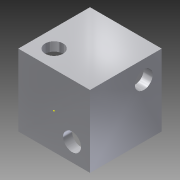
# Autodesk Inventor part: Corner
Saved by Autodesk Inventor 2015 SP1 (Build 190203100, 203)
## iProperties
Created: 2015-06-22
Part Number: Corner
Material: Aluminum 6061
Document SubType Name: Modeling
Designer: Kartikye
Density: 2.7 g/cm^3
Appearance: Aluminum - Flat
Author: Kartikye
Autodesk Inventor part; units mm, degrees
ref_plane "YZ Plane" through (0, 0, 0) normal (1, 0, 0) x (0, 1, 0)
ref_plane "XZ Plane" through (0, 0, 0) normal (0, 1, 0) x (-1, 0, 0)
ref_plane "XY Plane" through (0, 0, 0) normal (0, 0, 1) x (1, 0, 0)
sketch "Sketch1" plane through (0, 0, 0) normal (0, 1, 0) x (-1, 0, 0)
  point P0 (0, 0)
sketch "Sketch2" plane through (0, 0, 0) normal (0, 1, 0) x (-1, 0, 0)
  line L0 (-4, 4) -> (4, 4)
  line L1 (4, 4) -> (4, -4)
  line L2 (4, -4) -> (-4, -4)
  line L3 (-4, -4) -> (-4, 4)
  line L4 (-4, 4) -> (4, -4) construction
  line L5 (4, 4) -> (-4, -4) construction
  point P0 (0, 0)
  dimension "d0" = 8
  dimension "d1" = 8
  constraints: 12 end point, 2 midpoint, 2 parallel, 1 horizontal, 1 perpendicular
  measures "d0" distance of L1.end L2.end
  measures "d1" distance of L0.end L1.end
extrude "Extrusion1" add sketch "Sketch2" along normal blind 8
sketch "Sketch3" plane through (-4, 0, -4) normal (-1, 0, 0) x (0, 0, 1)
  line L0 (0, 1) -> (7, 1)
  line L1 (7, 1) -> (7, 7)
  line L2 (7, 7) -> (0, 7)
  line L3 (0, 7) -> (0, 1)
  line L4 (8, 0) -> (0, 0) projected
  line L5 (0, 0) -> (0, 8) projected
  point P0 (4, 0)
  dimension "d4" = 7
  dimension "d5" = 6
  dimension "d6" = 1
  dimension "d7" = 0
  constraints: 8 end point, 2 parallel, 1 horizontal, 1 perpendicular
  measures "d4" distance of L2.end L1.end
  measures "d5" distance of L1.end L0.end
  measures "d6" distance between parallel lines of L4 L0
  measures "d7" distance between parallel lines of L5 L3
extrude "Extrusion2" cut sketch "Sketch3" against normal blind 7
sketch "Sketch4" plane through (-4, 0, 4) normal (0, 0, 1) x (1, 0, 0)
  circle A0 centre (2, 2) radius 1
  line L0 (8, 0) -> (0, 0) projected
  line L1 (8, 0) -> (8, 8) projected
  point P0 (4, 0)
  dimension "d10" = 2
  dimension "d11" = 2
  dimension "d12" = 6
  constraints: 1 centre point
  measures "d10" diameter of A0
  measures "d11" distance from line of A0.centre L0
  measures "d12" distance from line of L1 A0.centre
sketch "Sketch5" plane through (4, 0, 4) normal (1, 0, 0) x (0, 0, -1)
  circle A0 centre (2, 6) radius 1
  line L0 (0, 0) -> (0, 8) projected
  line L1 (8, 0) -> (0, 0) projected
  point P0 (4, 0)
  dimension "d13" = 2
  dimension "d14" = 2
  dimension "d15" = 6
  constraints: 1 centre point
  measures "d13" diameter of A0
  measures "d14" distance from line of L0 A0.centre
  measures "d15" distance from line of L1 A0.centre
sketch "Sketch6" plane through (0, 0, 0) normal (0, -1, 0) x (1, 0, 0)
  circle A0 centre (2, -2) radius 1
  line L0 (4, 4) -> (-4, 4) projected
  line L1 (4, -4) -> (4, 4) projected
  point P0 (0, 0)
  dimension "d16" = 2
  dimension "d17" = 6
  dimension "d18" = 2
  constraints: 1 centre point
  measures "d16" diameter of A0
  measures "d17" distance from line of L0 A0.centre
  measures "d18" distance from line of L1 A0.centre
extrude "Extrusion3" cut sketch "Sketch6" against normal blind 1
extrude "Extrusion4" cut sketch "Sketch5" against normal blind 1
extrude "Extrusion5" cut sketch "Sketch4" against normal blind 1
sketch "Sketch7" plane through (0, 8, 0) normal (0, 1, 0) x (1, 0, 0)
  circle A0 centre (0, 0) radius 1
  line L0 (4, 4) -> (-4, 4) projected
  line L1 (-4, 4) -> (-4, -4) projected
  dimension "d25" = 2
  dimension "d26" = 4
  dimension "d27" = 4
  constraints: 1 centre point
  measures "d25" diameter of A0
  measures "d26" distance from line of A0.centre L0
  measures "d27" distance from line of L1 A0.centre
extrude "Extrusion6" cut sketch "Sketch7" against normal blind 1
body "Solid1"
